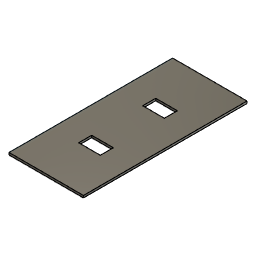
Bottom_PanleV2+v1 (Autodesk Fusion 360 archive; units mm, degrees)
design "Bottom cover v1"
Autodesk Fusion 360 part; units mm, degrees
sketch "Sketch1" plane through (0, 0, 0) normal (0, 1, 0) x (1, 0, 0)
  line L0 (0, 0) -> (170, 0)
  line L1 (170, 0) -> (170, -376)
  line L2 (170, -376) -> (0, -376)
  line L3 (0, -376) -> (0, 0)
  dimension "d1" = 170
  dimension "d2" = 376
  constraint horizontal L0
  constraint vertical L1
  constraint horizontal L2
  constraint vertical L3
  constraint coincident L0.start L3.end
  measures "d1" distance of L0.start L0.end
  measures "d2" distance of L0.start L2.end
extrude "Extrude1" add sketch "Sketch1" along normal blind 5
sketch "Sketch2" plane through (0, 0, 0) normal (-1, 0, 0) x (0, 0, 1)
  line L0 (0, 0) -> (376, 0)
  line L1 (376, 0) -> (376, 5)
  line L2 (376, 5) -> (0, 5)
  line L3 (0, 5) -> (0, 0)
extrude "Extrude2" cut 1 faces at (56.6667, 1.6667, 0) along direction (0, 0, 1) blind 3
extrude "Extrude3" cut 1 faces at (170, 1.6667, 127.3333) along direction (-1, 0, 0) blind 3
extrude "Extrude4" add 1 faces at (55.6667, 1.6667, 3) along direction (0, 0, -1) blind 3
extrude "Extrude5" add 1 faces at (167, 1.6667, 250.6667) along direction (1, 0, 0) blind 2
extrude "Extrude6" add 1 faces at (56.3333, 1.6667, 376) along direction (0, 0, 1) blind 2
extrude "Extrude7" add 1 faces at (169, 3.3333, 252) along direction (1, 0, 0) blind 3
sketch "Sketch3" plane through (0, 5, 0) normal (0, 1, 0) x (-1, 0, 0)
  line L0 (-172, 0) -> (0, 0)
  line L1 (0, 0) -> (0, 378)
  line L2 (0, 378) -> (-172, 378)
  line L3 (-172, 378) -> (-172, 0)
  line L4 (-61, 248) -> (-111, 248)
  line L5 (-111, 248) -> (-111, 278)
  line L6 (-111, 278) -> (-61, 278)
  line L7 (-61, 278) -> (-61, 248)
  line L8 (-61, 100) -> (-111, 100)
  line L9 (-111, 100) -> (-111, 130)
  line L10 (-111, 130) -> (-61, 130)
  line L11 (-61, 130) -> (-61, 100)
  dimension "d17" = 50
  dimension "d18" = 30
  dimension "d19" = 50
  dimension "d20" = 30
  dimension "d21" = 100
  dimension "d22" = 100
  dimension "d23" = 61
  dimension "d24" = 61
  constraint horizontal L4
  constraint vertical L5
  constraint horizontal L6
  constraint vertical L7
  constraint horizontal L8
  constraint vertical L9
  constraint horizontal L10
  constraint vertical L11
  measures "d17" distance of L4.start L4.end
  measures "d18" distance of L4.start L6.end
  measures "d19" distance of L8.start L8.end
  measures "d20" distance of L8.start L10.end
  measures "d21" vertical distance of L1.end L6.end
  measures "d22" vertical distance of L0.end L8.start
  measures "d23" horizontal distance of L1.end L6.end
  measures "d24" horizontal distance of L0.end L8.start
extrude "Extrude8" cut sketch "Sketch3" against normal blind 5 contours L4 L5 L6 L7 | L8 L9 L10 L11

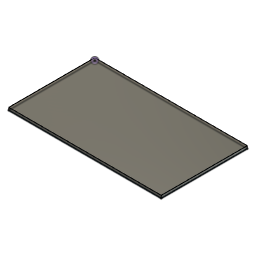
design "L&R_panel v2"
Autodesk Fusion 360 part; units mm, degrees
sketch "Sketch1" plane through (0, 0, 0) normal (0, 1, 0) x (1, 0, 0)
  line L0 (0, 0) -> (381, 0)
  line L1 (381, 0) -> (381, -215)
  line L2 (381, -215) -> (0, -215)
  line L3 (0, -215) -> (0, 0)
  dimension "d2" = 381
  dimension "d3" = 215
  constraint horizontal L0
  constraint vertical L1
  constraint horizontal L2
  constraint vertical L3
  constraint coincident L0.start L3.end
  measures "d2" distance of L0.start L0.end
  measures "d3" distance of L0.start L2.end
sketch "Sketch2" plane through (0, 0, 0) normal (0, 1, 0) x (1, 0, 0)
extrude "Extrude1" add sketch "Sketch1" along normal blind 6.35

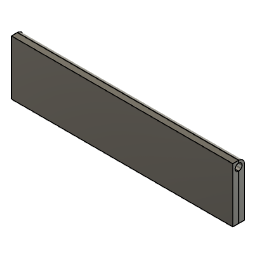
design "front bottom cover"
Autodesk Fusion 360 part; units mm, degrees
sketch "Sketch1" plane through (0, 0, 0) normal (0, 0, 1) x (1, 0, 0)
  line L0 (0, 0) -> (175, 0)
  line L1 (175, 0) -> (175, 46.35)
  line L2 (175, 46.35) -> (0, 46.35)
  line L3 (0, 46.35) -> (0, 0)
  dimension "d1" = 175
  dimension "d2" = 46.35
  constraint horizontal L0
  constraint vertical L1
  constraint horizontal L2
  constraint vertical L3
  constraint coincident L0.start L3.end
  measures "d1" distance of L0.start L0.end
  measures "d2" distance of L0.start L2.end
extrude "Extrude1" add sketch "Sketch1" along normal blind 8 makes body 1
extrude "Extrude2" add 1 faces at (58.3333, 30.9, 8) along direction (0, 0, 1) blind 2 on bodies 1 bodies 1
sketch "Sketch2" plane through (175, 0, 0) normal (1, 0, 0) x (0, 0, -1)
  line L0 (0, 0) -> (0, 46.35)
  line L1 (0, 46.35) -> (-10, 46.35)
  line L2 (-10, 46.35) -> (-10, 0)
  line L3 (-10, 0) -> (0, 0)
  circle A0 centre (-5, 41) radius 3
  dimension "d7" = 6
  measures "d7" diameter of A0
extrude "Extrude3" cut sketch "Sketch2" against normal blind 10 contours A0 bodies 1
sketch "Sketch3" plane through (0, 0, 0) normal (1, 0, 0) x (0, 0, -1)
sketch "Sketch4" plane through (0, 0, 0) normal (-1, 0, 0) x (0, 0, 1)
  line L0 (0, 46.35) -> (0, 0)
  line L1 (0, 0) -> (10, 0)
  line L2 (10, 0) -> (10, 46.35)
  line L3 (10, 46.35) -> (0, 46.35)
  circle A0 centre (5, 41) radius 3
  dimension "d10" = 6
  dimension "d11" = 5.35
  measures "d10" diameter of A0
  measures "d11" distance of L3 A0.centre
extrude "Extrude4" cut sketch "Sketch4" against normal blind 10 contours A0 bodies 1
sketch "Sketch5" plane through (0, 0, 0) normal (0, 0, 1) x (1, 0, 0)
sketch "Sketch6" plane through (0, 0, 0) normal (-1, 0, 0) x (0, 0, 1)
  circle A0 centre (5, 41) radius 3
  line L0 (0, 46.35) -> (0, 0)
  line L1 (0, 0) -> (10, 0)
  line L2 (10, 0) -> (10, 46.35)
  line L3 (10, 46.35) -> (0, 46.35)
  arc A1 (5, 46) -> (0, 41) centre (5, 41) ccw
  line L4 (5, 46) -> (10, 46)
  line L5 (0, 41) -> (0, 46.35)
  line L6 (10, 46.35) -> (0, 46.35)
  line L7 (10, 46.35) -> (10, 46)
  constraint concentric A0 A1
  constraint tangent L0 A1
  constraint coincident L0 A1.end
  constraint coincident L2 L4.end
  constraint tangent A1 L4
  constraint perpendicular L2 L4
  constraint coincident L0.start L3.end
  constraint coincident L2.end L3.start
extrude "Extrude5" cut sketch "Sketch6" against normal through all contours L0 L2 L3 A1 L4 L5 L6 L7 bodies 1
ref_plane "WorkPlane1" through (87.5, 23.175, 5) normal (0, 0, -1) x (-1, 0, 0)
extrude "Extrude6" add 2 faces at (58.3333, 0, 3.3333) (58.3333, 0, 3.3333) along direction (0, -1, 0) blind 0.381 on bodies 1 bodies 1
extrude "Extrude7" add 1 faces at (175, 12.4155, 4.9253) along direction (1, 0, 0) blind 12.7 on bodies 1 bodies 1
split "Split3" by plane through (87.5, 23.175, 5) normal (0, 0, -1) bodies 1 makes body 2 at (125.1333, 13.4127, 0)

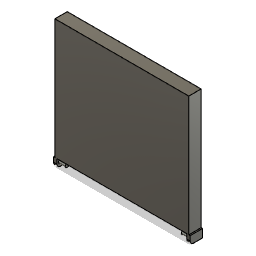
design "door"
Autodesk Fusion 360 part; units mm, degrees
sketch "Sketch1" plane through (0, 0, 0) normal (0, 0, 1) x (1, 0, 0)
  line L0 (-14, 0) -> (175, 0)
  line L1 (180, -12) -> (180, 0)
  line L2 (178, 175) -> (-17, 175)
  line L3 (-19, 0) -> (-19, -12)
  line L4 (-19, -12) -> (-14, -12)
  line L5 (-14, -12) -> (-14, 0)
  line L6 (180, -12) -> (175, -12)
  line L7 (175, -12) -> (175, 0)
  line L8 (180, 0) -> (178, 0)
  line L9 (178, 0) -> (178, 175)
  line L10 (-17, 0) -> (-17, 175)
  line L11 (-17, 0) -> (-19, 0)
  dimension "d1" = 189
  dimension "d13" = 12
  dimension "d14" = 12
  dimension "d16" = 5
  dimension "d24" = 175
  dimension "d31" = 2
  dimension "d32" = 5
  dimension "d33" = 2
  constraint horizontal L0
  constraint vertical L1
  constraint perpendicular L2 L3
  constraint perpendicular L3 L4
  constraint perpendicular L0 L5
  constraint perpendicular L1 L6
  constraint perpendicular L0 L7
  constraint coincident L1.end L8.start
  constraint perpendicular L1 L8
  constraint perpendicular L2 L9
  constraint perpendicular L2 L10
  constraint perpendicular L3 L11
  measures "d1" distance of L0.start L0.end
  measures "d13" distance of L0.end L6.end
  measures "d14" distance of L0.start L4.end
  measures "d16" distance of L1.start L6.end
  measures "d24" distance of L0 L2
  measures "d31" distance of L1.end L8.end
  measures "d32" distance of L3.end L4.end
  measures "d33" distance of L10.start L3.start
extrude "Extrude1" add sketch "Sketch1" along normal blind 10
sketch "Sketch2" plane through (-14, 0, 0) normal (1, 0, 0) x (0, 0, -1)
  line L0 (0, -12) -> (0, 0)
  line L1 (0, 0) -> (-10, 0)
  line L2 (-10, 0) -> (-10, -12)
  line L3 (-10, -12) -> (0, -12)
  circle A0 centre (-5, -5.6) radius 2.9
  dimension "d5" = 5.8
  dimension "d6" = 5.6
  measures "d5" diameter of A0
  measures "d6" distance of L1 A0.centre
extrude "Extrude2" add sketch "Sketch2" along normal blind 10 contours A0
sketch "Sketch3" plane through (175, 0, 0) normal (-1, 0, 0) x (0, 0, 1)
  line L0 (0, 0) -> (0, -12)
  line L1 (0, -12) -> (10, -12)
  line L2 (10, -12) -> (10, 0)
  line L3 (10, 0) -> (0, 0)
  circle A0 centre (5, -5.6) radius 2.9
  dimension "d9" = 5.8
  dimension "d10" = 5.6
  measures "d9" diameter of A0
  measures "d10" distance of L3 A0.centre
extrude "Extrude3" add sketch "Sketch3" along normal blind 10 contours A0
sketch "Sketch4" plane through (0, 0, 0) normal (0, 0, -1) x (-1, 0, 0)
  line L0 (19, -12) -> (19, 0)
  line L1 (17, 0) -> (17, 175)
  line L2 (17, 175) -> (-178, 175)
  line L3 (-178, 175) -> (-178, 0)
  line L4 (-178, 0) -> (-180, 0)
  line L5 (-180, 0) -> (-180, -12)
  line L6 (-180, -12) -> (-175, -12)
  line L7 (-175, -12) -> (-175, 0)
  line L8 (-175, 0) -> (14, 0)
  line L9 (14, 0) -> (14, -12)
  line L10 (14, -12) -> (19, -12)
  line L11 (-178, 0) -> (-180, 0)
  line L12 (-180, 0) -> (-180, -12)
  line L13 (-180, -12) -> (-175, -12)
  line L14 (-175, -12) -> (-175, 172)
  line L15 (-175, 172) -> (14, 172)
  line L16 (14, 172) -> (14, -12)
  line L17 (14, -12) -> (19, -12)
  line L18 (19, -12) -> (19, 0)
  line L19 (19, 0) -> (17, 0)
  line L20 (17, 0) -> (17, 175)
  line L21 (17, 175) -> (-178, 175)
  line L22 (-178, 175) -> (-178, 0)
  line L23 (19, 0) -> (17, 0)
  dimension "d19" = 3
  dimension "d20" = 3
  dimension "d21" = 3
  constraint coincident L3.end L4.start
  constraint coincident L4.end L5.start
  constraint coincident L5.end L6.start
  constraint coincident L6 L7.start
  constraint perpendicular L6 L14
  constraint perpendicular L3 L15
  constraint perpendicular L8 L16
  constraint coincident L10 L9.end
  constraint coincident L0.start L10.end
  constraint coincident L0.end L18.end
  constraint coincident L1.start L19.end
  constraint coincident L1.end L2.start
  constraint coincident L2.end L3.start
  measures "d19" distance of L16 L20
  measures "d20" distance of L14 L22
  measures "d21" distance of L15 L21
extrude "Extrude4" add sketch "Sketch4" along normal blind 8 contours L0 L1 L2 L3 L4 L5 L6 L7 L9 L10 L11 L12 L13 L14 L15 L16 L17 L18 L19 L20 L21 L22 L23
fillet "Fillet1" radius 5 1 edges at (-16.5, -12, 10)
fillet "Fillet2" radius 5 1 edges at (177.5, -12, 10)
extrude "Extrude5" cut 1 faces at (112, 114.6667, 0) along direction (0, 0, 1) blind 2

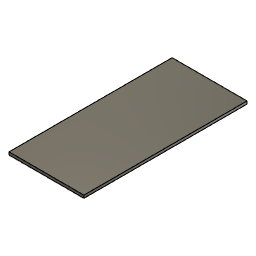
design "T_Panel v1"
Autodesk Fusion 360 part; units mm, degrees
sketch "Sketch1" plane through (0, 0, 0) normal (0, 1, 0) x (1, 0, 0)
  line L0 (0, 0) -> (175, 0)
  line L1 (175, 0) -> (175, -381)
  line L2 (175, -381) -> (0, -381)
  line L3 (0, -381) -> (0, 0)
  dimension "d1" = 175
  dimension "d2" = 381
  constraint horizontal L0
  constraint vertical L1
  constraint horizontal L2
  constraint vertical L3
  constraint coincident L0.start L3.end
  measures "d1" distance of L0.start L0.end
  measures "d2" distance of L0.start L2.end
extrude "Extrude1" add sketch "Sketch1" along normal blind 6.35
